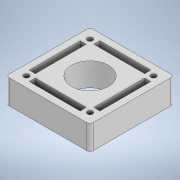
# Autodesk Inventor part: ShoulderMotorSupport
Saved by Autodesk Inventor 2022 (Build 260153000, 153)
## iProperties
Created: 2022-03-01
Part Number: ShoulderMotorSupport
Material: Genérico
Document SubType Name: Modeling
Designer: JK
Density: 1 g/cm^3
Appearance: Valor por defecto
Author: JK
Autodesk Inventor part; units mm, degrees
ref_plane "YZ Plane" through (0, 0, 0) normal (1, 0, 0) x (0, 1, 0)
ref_plane "XZ Plane" through (0, 0, 0) normal (0, 1, 0) x (-1, 0, 0)
ref_plane "XY Plane" through (0, 0, 0) normal (0, 0, 1) x (1, 0, 0)
sketch "Boceto1" plane through (0, 0, 0) normal (0, 1, 0) x (-1, 0, 0)
  circle A0 centre (0, 0) radius 18.15
  line L0 (-41.2, 41.2) -> (41.2, 41.2)
  line L1 (41.2, 41.2) -> (41.2, -41.2)
  line L2 (41.2, -41.2) -> (-41.2, -41.2)
  line L3 (-41.2, -41.2) -> (-41.2, 41.2)
  line L4 (-41.2, 41.2) -> (41.2, -41.2) construction
  line L5 (41.2, 41.2) -> (-41.2, -41.2) construction
  dimension "d0" = 36.3
  dimension "d1" = 82.4
  dimension "d2" = 82.4
  constraints: 12 end point, 2 midpoint, 2 parallel, 1 centre point, 1 coincident, 1 horizontal, 1 perpendicular
  measures "d0" diameter of A0
  measures "d1" distance of L0.end L1.end
  measures "d2" distance of L1.end L2.end
extrude "Extrusión1" add sketch "Boceto1" along normal blind 23
fillet "Empalme1" radius 3 4 edges at (-41.2, 11.5, 41.2) (41.2, 11.5, 41.2) (41.2, 11.5, -41.2) (-41.2, 11.5, -41.2)
sketch "Boceto3" plane through (0, 0, 0) normal (0, -1, 0) x (1, 0, 0)
  circle A0 centre (31.2, -31.2) radius 2.65
  line L0 (41.2, 38.2) -> (41.2, -38.2) projected
  line L1 (38.2, -41.2) -> (-38.2, -41.2) projected
  point P0 (0, 0)
  dimension "d10" = 5.3
  dimension "d11" = 10
  dimension "d12" = 10
  constraints: 1 centre point
  measures "d10" diameter of A0
  measures "d11" distance from line of L0 A0.centre
  measures "d12" distance from line of L1 A0.centre
extrude "Extrusión3" cut sketch "Boceto3" against normal through all
pattern_circular "Patrón circular1" count 4 over 360 about axis through (0, 0, 0) along (0, 1, 0) of "Extrusión3"
sketch "Boceto7" plane through (0, 0, 0) normal (0, -1, 0) x (1, 0, 0)
  line L0 (-21.2, -21.2) -> (21.2, -21.2)
  line L1 (21.2, -21.2) -> (21.2, 21.2)
  line L2 (21.2, 21.2) -> (-21.2, 21.2)
  line L3 (-21.2, 21.2) -> (-21.2, -21.2)
  line L4 (-21.2, -21.2) -> (21.2, 21.2) construction
  line L5 (21.2, -21.2) -> (-21.2, 21.2) construction
  circle A0 centre (31.2, 31.2) radius 2.65 projected
  line L6 (41.2, 110.8874) -> (21.2, -48.4874) construction
  line L7 (21.2, 110.8874) -> (41.2, -48.4874) construction
  circle A1 centre (31.2, 31.2) radius 2.65 projected
  circle A2 centre (-31.2, 31.2) radius 2.65 projected
  circle A3 centre (-31.2, -31.2) radius 2.65 projected
  circle A4 centre (31.2, -31.2) radius 2.65 projected
  arc A5 (-41.2, -38.2) -> (-38.2, -41.2) centre (-38.2, -38.2) ccw projected
  line L8 (38.2, -41.2) -> (-38.2, -41.2) projected
  arc A6 (38.2, -41.2) -> (41.2, -38.2) centre (38.2, -38.2) ccw projected
  line L9 (41.2, 38.2) -> (41.2, -38.2) projected
  arc A7 (41.2, 38.2) -> (38.2, 41.2) centre (38.2, 38.2) ccw projected
  line L10 (-38.2, 41.2) -> (38.2, 41.2) projected
  arc A8 (-38.2, 41.2) -> (-41.2, 38.2) centre (-38.2, 38.2) ccw projected
  line L11 (-41.2, -38.2) -> (-41.2, 38.2) projected
  circle A9 centre (0, 0) radius 18.15 projected
  dimension "d27" = 42.4
  dimension "d28" = 42.4
  dimension "d29" = 20
  constraints: 16 end point, 4 midpoint, 2 parallel, 1 horizontal, 1 perpendicular
  measures "d27" distance of L2.end L1.end
  measures "d28" distance of L1.end L0.end
  measures "d29" distance of L7.end L6.end
extrude "Extrusión5" add sketch "Boceto7" along normal blind 1 contours L11 A8 L10 A7 L9 A6 L8 A5
sketch "Boceto8" plane through (0, -1, 0) normal (0, -1, 0) x (1, 0, 0)
  line L0 (-34.7, -25) -> (-28.7, -25)
  line L1 (-28.7, -25) -> (-28.7, 25)
  line L2 (-28.7, 25) -> (-34.7, 25)
  line L3 (-34.7, 25) -> (-34.7, -25)
  line L4 (-34.7, -25) -> (-28.7, 25) construction
  line L5 (-28.7, -25) -> (-34.7, 25) construction
  point P0 (0, 0)
  point P1 (-31.7, 0)
  dimension "d32" = 6
  dimension "d33" = 50
  constraints: 12 end point, 2 midpoint, 2 parallel, 1 horizontal, 1 perpendicular
  measures "d32" distance of L2.end L1.end
  measures "d33" distance of L1.end L0.end
extrude "Extrusión6" cut sketch "Boceto8" against normal through all
pattern_circular "Patrón circular3" count 4 over 360 about axis through (0, 0, 0) along (0, 1, 0) of "Extrusión6"
sketch "Boceto5" plane through (0, 23, 0) normal (0, 1, 0) x (1, 0, 0)
  line L0 (27.934, -34.466) -> (26.7386, -30.0046)
  line L1 (26.7386, -30.0046) -> (30.0046, -26.7386)
  line L2 (30.0046, -26.7386) -> (34.466, -27.934)
  line L3 (34.466, -27.934) -> (35.6614, -32.3954)
  line L4 (35.6614, -32.3954) -> (32.3954, -35.6614)
  line L5 (32.3954, -35.6614) -> (27.934, -34.466)
  circle A0 centre (31.2, -31.2) radius 4
  line L6 (41.2, -38.2) -> (41.2, 38.2) projected
  circle A1 centre (31.2, -31.2) radius 2.65 projected
  point P0 (0, 0)
  dimension "d18" = 8
  dimension "d19" = 45
  dimension "d25" = 42.4
  dimension "d26" = 42.4
  constraints: 12 end point, 2 midpoint, 2 parallel, 1 horizontal, 1 perpendicular
  measures "d25" distance of L2.end L1.end
  measures "d26" distance of L1.end L0.end
